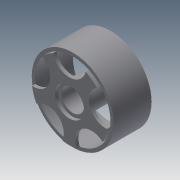
# Autodesk Inventor part: Wheel
Saved by Autodesk Inventor 2015 (Build 190159000, 159)
## iProperties
Created: 2016-11-06
Part Number: Wheel
Material: Generic
Document SubType Name: Modeling
Designer: Aniket Pant
Density: 1 g/cm^3
Appearance: Default
Author: Aniket Pant
Autodesk Inventor part; units mm, degrees
ref_plane "YZ Plane" through (0, 0, 0) normal (1, 0, 0) x (0, 1, 0)
ref_plane "XZ Plane" through (0, 0, 0) normal (0, 1, 0) x (-1, 0, 0)
ref_plane "XY Plane" through (0, 0, 0) normal (0, 0, 1) x (1, 0, 0)
sketch "Sketch1" plane through (0, 0, 0) normal (0, 0, 1) x (1, 0, 0)
  circle A0 centre (0, 0) radius 15.748
  circle A1 centre (0, 0) radius 14.478
  circle A2 centre (0, 0) radius 5.588
  circle A3 centre (0, 0) radius 4.318
  dimension "d0" = 1.27
  dimension "d1" = 8.89
  dimension "d2" = 1.27
  dimension "d3" = 11.176
  constraints: 4 centre point, 2 coincident
  measures "d0" radial gap between concentric circles of A0 A1
  measures "d1" radial gap between concentric circles of A2 A1
  measures "d2" radial gap between concentric circles of A3 A2
  measures "d3" diameter of A2
extrude "Extrusion1" add sketch "Sketch1" along normal blind 14.478
sketch "Sketch2" plane through (0, 0, 14.478) normal (0, 0, 1) x (1, 0, 0)
  circle A0 centre (0, 0) radius 14.478 projected
  circle A1 centre (0, 0) radius 15.748 projected
  circle A2 centre (0, 0) radius 4.318 projected
  circle A3 centre (0, 0) radius 5.588 projected
extrude "Extrusion2" add sketch "Sketch2" along normal blind 1.27 contours A0
sketch "Sketch3" plane through (0, 0, 15.748) normal (0, 0, 1) x (1, 0, 0)
  circle A0 centre (0, 0) radius 14.478 projected
  circle A1 centre (0, 0) radius 4.318 projected
  circle A2 centre (0, 0) radius 14.478 projected
  circle A3 centre (0, 0) radius 15.748 projected
  circle A4 centre (0, 0) radius 14.478 projected
  circle A5 centre (0, 0) radius 15.748 projected
  circle A6 centre (0, 0) radius 4.318 projected
  circle A7 centre (0, 0) radius 5.588 projected
  arc A8 (-6.1998, 13.0834) -> (6.1911, 13.0875) centre (-0.0048, 14.478) ccw
  dimension "d9" = 12.7
  constraints: 5 point on circle, 1 centre point, 2 other
  measures "d9" diameter of A8
extrude "Extrusion3" cut sketch "Sketch3" against normal up to next contours A8 A0 picked at (1.8159, 12.3862)
pattern_circular "Circular Pattern1" count 5 over 360 about axis through (0, 0, 14.478) along (0, 0, 1) of "Extrusion3"
body "Solid1"
